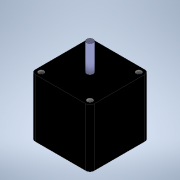
# Autodesk Inventor part: Motor Nema23
Saved by Autodesk Inventor 2021 (Build 250183000, 183)
## iProperties
Created: 2022-01-20
Part Number: Motor Nema23
Material: Generic
Document SubType Name: Modeling
Designer: deuts
Density: 1 g/cm^3
Appearance: Default
Author: deuts
Autodesk Inventor part; units mm, degrees
ref_plane "YZ Plane" through (0, 0, 0) normal (1, 0, 0) x (0, 1, 0)
ref_plane "XZ Plane" through (0, 0, 0) normal (0, 1, 0) x (-1, 0, 0)
ref_plane "XY Plane" through (0, 0, 0) normal (0, 0, 1) x (1, 0, 0)
sketch "Sketch1" plane through (0, 0, 0) normal (0, 1, 0) x (-1, 0, 0)
  line L0 (-28.5, 28.5) -> (28.5, 28.5)
  line L1 (28.5, 28.5) -> (28.5, -28.5)
  line L2 (28.5, -28.5) -> (-28.5, -28.5)
  line L3 (-28.5, -28.5) -> (-28.5, 28.5)
  line L4 (-28.5, 28.5) -> (28.5, -28.5) construction
  line L5 (28.5, 28.5) -> (-28.5, -28.5) construction
  point P0 (0, 0)
  dimension "d0" = 57
  dimension "d1" = 57
  constraints: 12 end point, 2 midpoint, 2 parallel, 1 horizontal, 1 perpendicular
  measures "d0" distance of L1.end L2.end
  measures "d1" distance of L0.end L1.end
extrude "Extrusion1" add sketch "Sketch1" along normal blind 56
sketch "Sketch2" plane through (0, 56, 0) normal (0, 1, 0) x (1, 0, 0)
  circle A0 centre (-23.57, 23.57) radius 2.6
  point P0 (0, 0)
  dimension "d6" = 5.2
  dimension "d19" = 23.57
  dimension "d20" = 23.57
  constraints: 1 centre point
  measures "d6" diameter of A0
  measures "d19" horizontal distance of point (0, 0) A0.centre
  measures "d20" horizontal distance of point (0, 0) A0.centre
extrude "Extrusion2" cut sketch "Sketch2" against normal blind 4.8
pattern_linear "Rectangular Pattern1" count 2 spacing 47.14 along (1, 0, 0) count 2 spacing 47.14 along (0, 0, 1) of "Extrusion2"
fillet "Fillet1" radius 4 4 edges at (28.5, 28, -28.5) (-28.5, 28, -28.5) (28.5, 28, 28.5) (-28.5, 28, 28.5)
sketch "Sketch3" plane through (0, 56, 0) normal (0, 1, 0) x (1, 0, 0)
  circle A0 centre (0, 0) radius 3.175
  dimension "d16" = 6.35
  constraints: 1 centre point, 1 coincident
  measures "d16" diameter of A0
extrude "Extrusion3" add sketch "Sketch3" along normal blind 26
body "Solid1"
